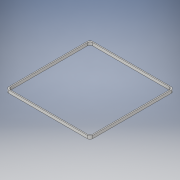
# Autodesk Inventor part: Coil5or6
Saved by Autodesk Inventor 2019 (Build 230136000, 136)
## iProperties
Created: 2021-05-17
Part Number: Coil5or6
Material: Generic
Document SubType Name: Modeling
Designer: jamieson-bl
Density: 1 g/cm^3
Appearance: Default
Author: jamieson-bl
Autodesk Inventor part; units mm, degrees
ref_plane "YZ Plane" through (0, 0, 0) normal (1, 0, 0) x (0, 1, 0)
ref_plane "XZ Plane" through (0, 0, 0) normal (0, 1, 0) x (-1, 0, 0)
ref_plane "XY Plane" through (0, 0, 0) normal (0, 0, 1) x (1, 0, 0)
sketch "Sketch1" plane through (0, 0, 0) normal (0, 1, 0) x (-1, 0, 0)
  line L0 (-950, -1020) -> (950, -1020)
  line L1 (1020, -950) -> (1020, 950)
  line L2 (950, 1020) -> (-950, 1020)
  line L3 (-1020, 950) -> (-1020, -950)
  line L4 (-1020, -1020) -> (1020, 1020) construction
  line L5 (1020, -1020) -> (-1020, 1020) construction
  line L6 (-925, -995) -> (925, -995)
  line L7 (995, -925) -> (995, 925)
  line L8 (925, 995) -> (-925, 995)
  line L9 (-995, 925) -> (-995, -925)
  line L10 (-995, -995) -> (995, 995) construction
  line L11 (995, -995) -> (-995, 995) construction
  arc A0 (995, 925) -> (925, 995) centre (925, 925) ccw
  arc A1 (1020, 950) -> (950, 1020) centre (950, 950) ccw
  arc A2 (925, -995) -> (995, -925) centre (925, -925) ccw
  arc A3 (950, -1020) -> (1020, -950) centre (950, -950) ccw
  arc A4 (-995, -925) -> (-925, -995) centre (-925, -925) ccw
  arc A5 (-1020, -950) -> (-950, -1020) centre (-950, -950) ccw
  arc A6 (-925, 995) -> (-995, 925) centre (-925, 925) ccw
  arc A7 (-950, 1020) -> (-1020, 950) centre (-950, 950) ccw
  point P0 (0, 0)
  dimension "d0" = 2040
  dimension "d1" = 2040
  dimension "d2" = 1990
  dimension "d3" = 1990
  dimension "d4" = 70
  constraints: 24 end point, 16 point on circle, 16 point on line, 16 tangent, 8 centre point, 7 equal radius, 4 midpoint, 4 parallel, 2 horizontal, 2 perpendicular
  measures "d0" distance of L5.end L4.end
  measures "d1" distance of L4.end L5.start
  measures "d2" distance of L11.end L10.end
  measures "d3" distance of L10.end L11.start
  measures "d4" radius of A0
extrude "Extrusion1" add sketch "Sketch1" along normal blind 70
body "Solid1"
